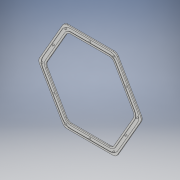
# Autodesk Inventor part: Flat Placeholder v1 - 175 - 12mm rim
Saved by Autodesk Inventor 2019 (Build 230136000, 136)
## iProperties
Created: 2021-07-14
Part Number: Flat Placeholder v1 - 175 - 12mm rim
Material: Generic
Document SubType Name: Modeling
Designer: Lix
Density: 1 g/cm^3
Appearance: Default
Author: Lix
## iProperties of the stored document Flat Placeholder v1 - 175 - 12mm rim - B_3DPrint.ipt
Created: 2021-08-07
Part Number: Flat Placeholder v1 - 175 - 12mm rim - B_3DPrint
Material: Generic
Document SubType Name: Modeling
Designer: Lix
Density: 1 g/cm^3
Appearance: Default
Author: Lix
Autodesk Inventor part; units mm, degrees
ref_plane "YZ Plane" through (0, 0, 0) normal (1, 0, 0) x (0, 1, 0)
ref_plane "XZ Plane" through (0, 0, 0) normal (0, 1, 0) x (-1, 0, 0)
ref_plane "XY Plane" through (0, 0, 0) normal (0, 0, 1) x (1, 0, 0)
sketch "Sketch1" plane through (0, 0, 0) normal (0, 0, 1) x (1, 0, 0)
  line L0 (50.5181, -87.5) -> (-50.5181, -87.5)
  line L1 (-50.5181, -87.5) -> (-101.0363, 0)
  line L2 (-101.0363, 0) -> (-50.5181, 87.5)
  line L3 (-50.5181, 87.5) -> (50.5181, 87.5)
  line L4 (50.5181, 87.5) -> (101.0363, 0)
  line L5 (101.0363, 0) -> (50.5181, -87.5)
  point P0 (0, 0)
  point P1 (0, 0)
  dimension "d0" = 175
  constraints: 12 end point, 1 coincident, 1 horizontal, 13 other
  measures "d0" distance between parallel lines of L4 L1
extrude "Extrusion1" add sketch "Sketch1" along normal blind 2
sketch "Sketch7" plane through (0, 0, 2) normal (0, 0, 1) x (1, 0, 0)
  line L0 (-50.5181, -87.5) -> (50.5181, -87.5) projected
  line L1 (50.5181, -87.5) -> (101.0363, 0) projected
  line L2 (101.0363, 0) -> (50.5181, 87.5) projected
  line L3 (50.5181, 87.5) -> (-50.5181, 87.5) projected
  line L4 (-50.5181, 87.5) -> (-101.0363, 0) projected
  line L5 (-101.0363, 0) -> (-50.5181, -87.5) projected
  line L6 (-43.5899, 75.5) -> (43.5899, 75.5)
  line L7 (43.5899, 75.5) -> (87.1799, 0)
  line L8 (87.1799, 0) -> (43.5899, -75.5)
  line L9 (43.5899, -75.5) -> (-43.5899, -75.5)
  line L10 (-43.5899, -75.5) -> (-87.1799, 0)
  line L11 (-87.1799, 0) -> (-43.5899, 75.5)
  dimension "d26" = 12
  constraints: 12 end point, 5 other
  measures "d26" distance between parallel lines of L3 L6
extrude "Extrusion6" cut sketch "Sketch7" against normal blind 7 contours L6 L7 L8 L9 L10 L11
fillet "Fillet2" radius 10 6 edges at (-87.1799, 0, 1) (-43.5899, -75.5, 1) (43.5899, -75.5, 1) (87.1799, 0, 1) (43.5899, 75.5, 1) (-43.5899, 75.5, 1)
fillet "Fillet3" radius 10 6 edges at (-50.5181, 87.5, 1) (50.5181, 87.5, 1) (101.0363, 0, 1) (50.5181, -87.5, 1) (-50.5181, -87.5, 1) (-101.0363, 0, 1)
sketch "Sketch9" plane through (0, 0, 2) normal (0, 0, 1) x (1, 0, 0)
  arc A0 (-98.1495, 5) -> (-98.1495, -5) centre (-89.4893, 0) ccw projected
  line L0 (-98.1495, -5) -> (-53.4049, -82.5) projected
  arc A1 (-53.4049, -82.5) -> (-44.7446, -87.5) centre (-44.7446, -77.5) ccw projected
  line L1 (-44.7446, -87.5) -> (44.7446, -87.5) projected
  arc A2 (44.7446, -87.5) -> (53.4049, -82.5) centre (44.7446, -77.5) ccw projected
  line L2 (53.4049, -82.5) -> (98.1495, -5) projected
  arc A3 (98.1495, -5) -> (98.1495, 5) centre (89.4893, 0) ccw projected
  line L3 (98.1495, 5) -> (53.4049, 82.5) projected
  arc A4 (53.4049, 82.5) -> (44.7446, 87.5) centre (44.7446, 77.5) ccw projected
  line L4 (44.7446, 87.5) -> (-44.7446, 87.5) projected
  arc A5 (-44.7446, 87.5) -> (-53.4049, 82.5) centre (-44.7446, 77.5) ccw projected
  line L5 (-53.4049, 82.5) -> (-98.1495, 5) projected
  line L6 (-84.2931, 5) -> (-46.4767, 70.5) projected
  arc A6 (-37.8164, 75.5) -> (-46.4767, 70.5) centre (-37.8164, 65.5) ccw projected
  line L7 (-37.8164, 75.5) -> (37.8164, 75.5) projected
  arc A7 (46.4767, 70.5) -> (37.8164, 75.5) centre (37.8164, 65.5) ccw projected
  line L8 (46.4767, 70.5) -> (84.2931, 5) projected
  arc A8 (84.2931, -5) -> (84.2931, 5) centre (75.6329, 0) ccw projected
  line L9 (84.2931, -5) -> (46.4767, -70.5) projected
  arc A9 (37.8164, -75.5) -> (46.4767, -70.5) centre (37.8164, -65.5) ccw projected
  line L10 (37.8164, -75.5) -> (-37.8164, -75.5) projected
  arc A10 (-46.4767, -70.5) -> (-37.8164, -75.5) centre (-37.8164, -65.5) ccw projected
  line L11 (-46.4767, -70.5) -> (-84.2931, -5) projected
  arc A11 (-84.2931, 5) -> (-84.2931, -5) centre (-75.6329, 0) ccw projected
  line L12 (-85.6329, 0) -> (-99.4893, 0) construction
  line L13 (-75.7772, 43.75) -> (-65.3849, 37.75) construction
  line L14 (-84.2931, 5) -> (-46.4767, 70.5) projected
  circle A12 centre (0, 81.5) radius 1.5
  circle A13 centre (-70.5811, 40.75) radius 1.5
  circle A14 centre (-92.5611, 0) radius 1.5
  circle A15 centre (70.5811, 40.75) radius 1.5
  circle A16 centre (0, 81.5) radius 1.5
  circle A17 centre (-46.2805, 80.1603) radius 1.5
  circle A18 centre (70.5811, -40.75) radius 1.5
  circle A19 centre (70.5811, 40.75) radius 1.5
  circle A20 centre (46.2805, 80.1603) radius 1.5
  circle A21 centre (0, -81.5) radius 1.5
  circle A22 centre (70.5811, -40.75) radius 1.5
  circle A23 centre (92.5611, 0) radius 1.5
  circle A24 centre (-70.5811, -40.75) radius 1.5
  circle A25 centre (0, -81.5) radius 1.5
  circle A26 centre (46.2805, -80.1603) radius 1.5
  circle A27 centre (-70.5811, 40.75) radius 1.5
  circle A28 centre (-70.5811, -40.75) radius 1.5
  circle A29 centre (-46.2805, -80.1603) radius 1.5
  point P0 (0, 0)
  point P1 (-70.5811, 40.75)
  dimension "d44" = 3
  dimension "d58" = 360
  constraints: 18 centre point, 7 coincident, 4 end point, 4 midpoint, 2 equal radius, 2 point on circle, 43 other
  measures "d44" diameter of A12
extrude "Extrusion8" add sketch "Sketch9" along normal blind 2 draft -10 contours A12 | A13 | A14 | A15 | A17 | A18 | A20 | A21 | A23 | A24 | A26 | A29
sketch "Sketch10" plane through (0, 0, 2) normal (0, 0, 1) x (1, 0, 0)
  arc A0 (-98.1495, 5) -> (-98.1495, -5) centre (-89.4893, 0) ccw projected
  line L0 (-98.1495, -5) -> (-53.4049, -82.5) projected
  arc A1 (-53.4049, -82.5) -> (-44.7446, -87.5) centre (-44.7446, -77.5) ccw projected
  line L1 (-44.7446, -87.5) -> (44.7446, -87.5) projected
  arc A2 (44.7446, -87.5) -> (53.4049, -82.5) centre (44.7446, -77.5) ccw projected
  line L2 (53.4049, -82.5) -> (98.1495, -5) projected
  arc A3 (98.1495, -5) -> (98.1495, 5) centre (89.4893, 0) ccw projected
  line L3 (98.1495, 5) -> (53.4049, 82.5) projected
  arc A4 (53.4049, 82.5) -> (44.7446, 87.5) centre (44.7446, 77.5) ccw projected
  line L4 (44.7446, 87.5) -> (-44.7446, 87.5) projected
  arc A5 (-44.7446, 87.5) -> (-53.4049, 82.5) centre (-44.7446, 77.5) ccw projected
  line L5 (-53.4049, 82.5) -> (-98.1495, 5) projected
  line L6 (-84.2931, 5) -> (-46.4767, 70.5) projected
  arc A6 (-37.8164, 75.5) -> (-46.4767, 70.5) centre (-37.8164, 65.5) ccw projected
  line L7 (-37.8164, 75.5) -> (37.8164, 75.5) projected
  arc A7 (46.4767, 70.5) -> (37.8164, 75.5) centre (37.8164, 65.5) ccw projected
  line L8 (46.4767, 70.5) -> (84.2931, 5) projected
  arc A8 (84.2931, -5) -> (84.2931, 5) centre (75.6329, 0) ccw projected
  line L9 (84.2931, -5) -> (46.4767, -70.5) projected
  arc A9 (37.8164, -75.5) -> (46.4767, -70.5) centre (37.8164, -65.5) ccw projected
  line L10 (37.8164, -75.5) -> (-37.8164, -75.5) projected
  arc A10 (-46.4767, -70.5) -> (-37.8164, -75.5) centre (-37.8164, -65.5) ccw projected
  line L11 (-46.4767, -70.5) -> (-84.2931, -5) projected
  arc A11 (-84.2931, 5) -> (-84.2931, -5) centre (-75.6329, 0) ccw projected
  line L12 (37.8164, 78.5) -> (-37.8164, 78.5)
  arc A12 (-37.8164, 78.5) -> (-49.0748, 72) centre (-37.8164, 65.5) ccw
  line L13 (-49.0748, 72) -> (-86.8912, 6.5)
  arc A13 (-86.8912, 6.5) -> (-86.8912, -6.5) centre (-75.6329, 0) ccw
  line L14 (-86.8912, -6.5) -> (-49.0748, -72)
  arc A14 (-49.0748, -72) -> (-37.8164, -78.5) centre (-37.8164, -65.5) ccw
  line L15 (-37.8164, -78.5) -> (37.8164, -78.5)
  arc A15 (37.8164, -78.5) -> (49.0748, -72) centre (37.8164, -65.5) ccw
  line L16 (49.0748, -72) -> (86.8912, -6.5)
  arc A16 (86.8912, -6.5) -> (86.8912, 6.5) centre (75.6329, 0) ccw
  line L17 (86.8912, 6.5) -> (49.0748, 72)
  arc A17 (49.0748, 72) -> (37.8164, 78.5) centre (37.8164, 65.5) ccw
  line L18 (-37.8164, 84.5) -> (37.8164, 84.5)
  arc A18 (54.2709, 75) -> (37.8164, 84.5) centre (37.8164, 65.5) ccw
  line L19 (54.2709, 75) -> (92.0874, 9.5)
  arc A19 (92.0874, -9.5) -> (92.0874, 9.5) centre (75.6329, 0) ccw
  line L20 (92.0874, -9.5) -> (54.2709, -75)
  arc A20 (37.8164, -84.5) -> (54.2709, -75) centre (37.8164, -65.5) ccw
  line L21 (37.8164, -84.5) -> (-37.8164, -84.5)
  arc A21 (-54.2709, -75) -> (-37.8164, -84.5) centre (-37.8164, -65.5) ccw
  line L22 (-54.2709, -75) -> (-92.0874, -9.5)
  arc A22 (-92.0874, 9.5) -> (-92.0874, -9.5) centre (-75.6329, 0) ccw
  line L23 (-92.0874, 9.5) -> (-54.2709, 75)
  arc A23 (-37.8164, 84.5) -> (-54.2709, 75) centre (-37.8164, 65.5) ccw
  point P0 (0, 0)
  dimension "d52" = 3
  dimension "d53" = 6
  constraints: 24 end point, 24 point on circle, 12 centre point, 22 other
  measures "d52" distance between parallel lines of L7 L12
  measures "d53" distance between parallel lines of L12 L18
extrude "Extrusion9" cut sketch "Sketch10" against normal blind 0.7 contours L18 A18 L19 A19 L20 A20 L21 A21 L22 A22 L23 A23
body "Solid1"
